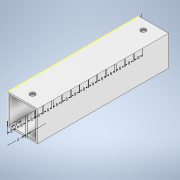
# Autodesk Inventor part: Cablecanal Ranurado 30 x 30 L=97
Saved by Autodesk Inventor 2020 (Build 240168000, 168)
## iProperties
Created: 2020-09-30
Part Number: Cablecanal Ranurado 30 x 30 L=97
Material: PVC-Piping
Document SubType Name: Modeling
Designer: Hernan
Density: 1.4 g/cm^3
Appearance: Smooth - White
Author: Hernan
Autodesk Inventor part; units mm, degrees
ref_plane "YZ Plane" through (0, 0, 0) normal (1, 0, 0) x (0, 1, 0)
ref_plane "XZ Plane" through (0, 0, 0) normal (0, 1, 0) x (-1, 0, 0)
ref_plane "XY Plane" through (0, 0, 0) normal (0, 0, 1) x (1, 0, 0)
sketch "Sketch1" plane through (0, 0, 0) normal (0, 0, 1) x (1, 0, 0)
  line L0 (-31.9903, -7.2804) -> (-1.9903, -7.2804)
  line L1 (-1.9903, -7.2804) -> (-1.9903, 22.7196)
  line L2 (-1.9903, 22.7196) -> (-31.9903, 22.7196)
  line L3 (-31.9903, -7.2804) -> (-31.9903, 22.7196)
  line L4 (-30.2903, 22.7196) -> (-30.2903, -7.2804)
  line L5 (-31.9903, -5.5804) -> (-1.9903, -5.5804)
  line L6 (-3.6903, 22.7196) -> (-3.6903, -7.2804)
  line L7 (-31.9903, 21.0196) -> (-1.9903, 21.0196)
  point P0 (0, 0)
  point P1 (0, 0)
  point P2 (-3.6903, 21.0196)
  point P3 (-30.2903, 21.0196)
  point P4 (-30.2903, -5.5804)
  point P5 (-3.6903, -5.5804)
  dimension "d0" = 30
  dimension "d1" = 30
  dimension "d2" = 1.7
  dimension "d3" = 1.7
  dimension "d4" = 1.7
  dimension "d5" = 1.7
  constraints: 16 end point, 8 point on line, 3 horizontal, 2 perpendicular, 2 vertical, 1 parallel
  measures "d0" distance of L0.start L0.end
  measures "d1" distance of L0.end L1.end
  measures "d2" distance between parallel lines of L0 L5
  measures "d3" distance between parallel lines of L3 L4
  measures "d4" distance between parallel lines of L1 L6
  measures "d5" distance between parallel lines of L2 L7
extrude "Extrusion1" add sketch "Sketch1" against normal blind 130
extrude "Extrusion2" cut sketch "Sketch1" against normal blind 130 contours L4 L7 L6 L5
sketch "Boceto2" plane through (-31.9903, 22.7196, 0) normal (0, 1, 0) x (1, 0, 0)
  line L0 (28.3, 130) -> (1.7, 130) projected
  line L1 (0, 0) -> (30, 0) projected
  circle A0 centre (15, 120) radius 2.5
  circle A1 centre (15, 10) radius 2.5
  line L2 (30, 0) -> (30, 130) projected
  point P0 (31.9903, 0)
  dimension "d12" = 5
  dimension "d13" = 5
  dimension "d14" = 110
  dimension "d15" = 10
  dimension "d16" = 15
  dimension "d17" = 15
  constraints: 2 centre point
  measures "d12" diameter of A0
  measures "d13" diameter of A1
  measures "d14" distance of A1.centre A0.centre
  measures "d15" distance from line of L1 A1.centre
  measures "d16" distance from line of L2 A0.centre
  measures "d17" distance from line of L2 A1.centre
extrude "Extrusión3" cut sketch "Boceto2" against normal blind 10
sketch "Boceto3" plane through (-31.9903, -7.2804, 0) normal (-1, 0, 0) x (0, 0, 1)
  line L0 (0, 0) -> (-8, 0)
  line L1 (0, 0) -> (-130, 0) projected
  line L2 (-8, 0) -> (-8, 5)
  line L3 (0, 0) -> (0, 5)
  line L4 (0, 30) -> (0, 0) projected
  line L5 (-1, 6.5) -> (-1, 30)
  line L6 (0, 30) -> (-130, 30) projected
  line L7 (-7, 6.5) -> (-7, 30)
  line L8 (-8, 5) -> (-7, 6.5)
  line L9 (-1, 6.5) -> (0, 5)
  line L10 (-10, 0) -> (-18, 0)
  line L11 (-18, 0) -> (-18, 5)
  line L12 (-10, 0) -> (-10, 5)
  line L13 (-11, 6.5) -> (-11, 30)
  line L14 (-17, 6.5) -> (-17, 30)
  line L15 (-18, 5) -> (-17, 6.5)
  line L16 (-11, 6.5) -> (-10, 5)
  line L17 (-20, 0) -> (-28, 0)
  line L18 (-28, 0) -> (-28, 5)
  line L19 (-20, 0) -> (-20, 5)
  line L20 (-21, 6.5) -> (-21, 30)
  line L21 (-27, 6.5) -> (-27, 30)
  line L22 (-28, 5) -> (-27, 6.5)
  line L23 (-21, 6.5) -> (-20, 5)
  line L24 (-27.0902, 0) -> (-35.0902, 0)
  line L25 (-35.0902, 0) -> (-35.0902, 5)
  line L26 (-27.0902, 0) -> (-27.0902, 5)
  line L27 (-28.0902, 6.5) -> (-28.0902, 30)
  line L28 (-34.0902, 6.5) -> (-34.0902, 30)
  line L29 (-35.0902, 5) -> (-34.0902, 6.5)
  line L30 (-28.0902, 6.5) -> (-27.0902, 5)
  line L31 (-36.249, 0) -> (-44.249, 0)
  line L32 (-44.249, 0) -> (-44.249, 5)
  line L33 (-36.249, 0) -> (-36.249, 5)
  line L34 (-37.249, 6.5) -> (-37.249, 30)
  line L35 (-43.249, 6.5) -> (-43.249, 30)
  line L36 (-44.249, 5) -> (-43.249, 6.5)
  line L37 (-37.249, 6.5) -> (-36.249, 5)
  line L38 (-45.3382, 0) -> (-53.3382, 0)
  line L39 (-53.3382, 0) -> (-53.3382, 5)
  line L40 (-45.3382, 0) -> (-45.3382, 5)
  line L41 (-46.3382, 6.5) -> (-46.3382, 30)
  line L42 (-52.3382, 6.5) -> (-52.3382, 30)
  line L43 (-53.3382, 5) -> (-52.3382, 6.5)
  line L44 (-46.3382, 6.5) -> (-45.3382, 5)
  line L45 (-54.7408, 0) -> (-62.7408, 0)
  line L46 (-62.7408, 0) -> (-62.7408, 5)
  line L47 (-54.7408, 0) -> (-54.7408, 5)
  line L48 (-55.7408, 6.5) -> (-55.7408, 30)
  line L49 (-61.7408, 6.5) -> (-61.7408, 30)
  line L50 (-62.7408, 5) -> (-61.7408, 6.5)
  line L51 (-55.7408, 6.5) -> (-54.7408, 5)
  line L52 (-63.4121, 0) -> (-71.4121, 0)
  line L53 (-71.4121, 0) -> (-71.4121, 5)
  line L54 (-63.4121, 0) -> (-63.4121, 5)
  line L55 (-64.4121, 6.5) -> (-64.4121, 30)
  line L56 (-70.4121, 6.5) -> (-70.4121, 30)
  line L57 (-71.4121, 5) -> (-70.4121, 6.5)
  line L58 (-64.4121, 6.5) -> (-63.4121, 5)
  line L59 (-72.0834, 0) -> (-80.0834, 0)
  line L60 (-80.0834, 0) -> (-80.0834, 5)
  line L61 (-72.0834, 0) -> (-72.0834, 5)
  line L62 (-73.0834, 6.5) -> (-73.0834, 30)
  line L63 (-79.0834, 6.5) -> (-79.0834, 30)
  line L64 (-80.0834, 5) -> (-79.0834, 6.5)
  line L65 (-73.0834, 6.5) -> (-72.0834, 5)
  line L66 (-80.9637, 0) -> (-88.9637, 0)
  line L67 (-88.9637, 0) -> (-88.9637, 5)
  line L68 (-80.9637, 0) -> (-80.9637, 5)
  line L69 (-81.9637, 6.5) -> (-81.9637, 30)
  line L70 (-87.9637, 6.5) -> (-87.9637, 30)
  line L71 (-88.9637, 5) -> (-87.9637, 6.5)
  line L72 (-81.9637, 6.5) -> (-80.9637, 5)
  line L73 (-89.8787, 0) -> (-97.8787, 0)
  line L74 (-97.8787, 0) -> (-97.8787, 5)
  line L75 (-89.8787, 0) -> (-89.8787, 5)
  line L76 (-90.8787, 6.5) -> (-90.8787, 30)
  line L77 (-96.8787, 6.5) -> (-96.8787, 30)
  line L78 (-97.8787, 5) -> (-96.8787, 6.5)
  line L79 (-90.8787, 6.5) -> (-89.8787, 5)
  line L80 (-98.7938, 0) -> (-106.7938, 0)
  line L81 (-106.7938, 0) -> (-106.7938, 5)
  line L82 (-98.7938, 0) -> (-98.7938, 5)
  line L83 (-99.7938, 6.5) -> (-99.7938, 30)
  line L84 (-105.7938, 6.5) -> (-105.7938, 30)
  line L85 (-106.7938, 5) -> (-105.7938, 6.5)
  line L86 (-99.7938, 6.5) -> (-98.7938, 5)
  line L87 (-107.8481, 0) -> (-115.8481, 0)
  line L88 (-115.8481, 0) -> (-115.8481, 5)
  line L89 (-107.8481, 0) -> (-107.8481, 5)
  line L90 (-108.8481, 6.5) -> (-108.8481, 30)
  line L91 (-114.8481, 6.5) -> (-114.8481, 30)
  line L92 (-115.8481, 5) -> (-114.8481, 6.5)
  line L93 (-108.8481, 6.5) -> (-107.8481, 5)
  line L94 (-116.8328, 0) -> (-124.8328, 0)
  line L95 (-124.8328, 0) -> (-124.8328, 5)
  line L96 (-116.8328, 0) -> (-116.8328, 5)
  line L97 (-117.8328, 6.5) -> (-117.8328, 30)
  line L98 (-123.8328, 6.5) -> (-123.8328, 30)
  line L99 (-124.8328, 5) -> (-123.8328, 6.5)
  line L100 (-117.8328, 6.5) -> (-116.8328, 5)
  line L101 (-126.0613, 0) -> (-134.0613, 0)
  line L102 (-134.0613, 0) -> (-134.0613, 5)
  line L103 (-126.0613, 0) -> (-126.0613, 5)
  line L104 (-127.0613, 6.5) -> (-127.0613, 30)
  line L105 (-133.0613, 6.5) -> (-133.0613, 30)
  line L106 (-134.0613, 5) -> (-133.0613, 6.5)
  line L107 (-127.0613, 6.5) -> (-126.0613, 5)
  point P0 (0, 7.2804)
  dimension "d20" = 8
  dimension "d26" = 8
  dimension "d27" = 8
  dimension "d28" = 8
  dimension "d29" = 8
  dimension "d30" = 8
  dimension "d31" = 8
  dimension "d32" = 8
  dimension "d33" = 8
  dimension "d34" = 8
  dimension "d35" = 8
  dimension "d36" = 8
  dimension "d37" = 8
  dimension "d38" = 8
  dimension "d39" = 8
  dimension "d40" = 2
  dimension "d41" = 2
  constraints: 210 end point, 4 point on line, 2 perpendicular
  measures "d20" distance of L0.start L0.end
  measures "d26" distance of L12.start L11.start
  measures "d27" distance of L19.start L18.start
  measures "d28" distance of L26.start L25.start
  measures "d29" distance of L33.start L32.start
  measures "d30" distance of L40.start L39.start
  measures "d31" distance of L47.start L46.start
  measures "d32" distance of L54.start L53.start
  measures "d33" distance of L61.start L60.start
  measures "d34" distance of L68.start L67.start
  measures "d35" distance of L75.start L74.start
  measures "d36" distance of L82.start L81.start
  measures "d37" distance of L89.start L88.start
  measures "d38" distance of L96.start L95.start
  measures "d39" distance of L103.start L102.start
  measures "d40" distance of L12.start L0.end
  measures "d41" distance of L19.start L11.start
body "Solid1"
